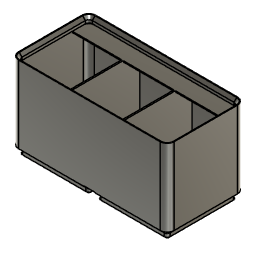
ForAnythingElse (Autodesk Fusion 360 design; units mm, degrees)
Autodesk Fusion 360 part; units mm, degrees
note: some values were not read from the file. Set by a fixed rule: which sketch regions a step uses.
ref_plane "WorkPlane9" through (0, 0, 5) normal (0, 0, 1) x (1, 0, 0)
ref_plane "WorkPlane10" through (21, 0, 0) normal (1, 0, 0) x (0, 1, 0)
ref_plane "WorkPlane11" through (0, 0, 42) normal (0, 0, 1) x (1, 0, 0)
sketch "BlockBaseProfle" plane through (0, 0, 0) normal (0, 0, 1) x (1, 0, 0)
  line L0 (0, 42) -> (42, 42)
  line L1 (42, 42) -> (42, 0)
  line L2 (42, 0) -> (0, 0)
  line L3 (0, 0) -> (0, 42)
  line L4 (0, 42) -> (42, 0) construction
  circle A0 centre (8, 8) radius 3.25
  circle A1 centre (8, 8) radius 1.5
  circle A2 centre (34, 8) radius 3.25
  circle A3 centre (34, 8) radius 1.5
  circle A4 centre (34, 34) radius 3.25
  circle A5 centre (34, 34) radius 1.5
  circle A6 centre (8, 34) radius 3.25
  circle A7 centre (8, 34) radius 1.5
  line L5 (11, 31) -> (31, 31)
  line L6 (31, 31) -> (31, 11)
  line L7 (31, 11) -> (11, 11)
  line L8 (11, 11) -> (11, 31)
  line L9 (11, 11) -> (31, 31) construction
  line L10 (4, 41.75) -> (38, 41.75)
  line L11 (41.75, 38) -> (41.75, 4)
  line L12 (38, 0.25) -> (4, 0.25)
  line L13 (0.25, 4) -> (0.25, 38)
  line L14 (21, 41.75) -> (21, 0.25) construction
  arc A8 (4, 41.75) -> (0.25, 38) centre (4, 38) ccw
  arc A9 (41.75, 38) -> (38, 41.75) centre (38, 38) ccw
  arc A10 (38, 0.25) -> (41.75, 4) centre (38, 4) ccw
  arc A11 (0.25, 4) -> (4, 0.25) centre (4, 4) ccw
  line L15 (0.25, 21) -> (41.75, 21) construction
  point P0 (21, 21)
  point P1 (21, 0.25)
  point P2 (21, 41.75)
  point P3 (0.25, 21)
  point P4 (41.75, 21)
  dimension "d8" = 42
  dimension "d11" = 8
  dimension "d12" = 8
  dimension "d13" = 6.5
  dimension "d14" = 3
  dimension "d16" = 360
  dimension "d24" = 20
  dimension "d30" = 0.25
  dimension "d31" = 3.75
  dimension "d34" = 0.25
  constraint horizontal L0
  constraint vertical L1
  constraint horizontal L2
  constraint vertical L3
  constraint equal L2 L3
  constraint midpoint L4 P0
  constraint coincident L2.end L3.start
  constraint concentric A0 A1
  constraint horizontal L5
  constraint vertical L6
  constraint horizontal L7
  constraint vertical L8
  constraint coincident L4 L6.end
  constraint coincident L4 L5.start
  constraint midpoint P0 L9
  constraint horizontal L10
  constraint vertical L11
  constraint horizontal L12
  constraint vertical L13
  constraint coincident P0 L14
  constraint coincident L10 P2
  constraint tangent L10 A8
  constraint tangent L13 A8
  constraint tangent L10 A9
  constraint tangent L11 A9
  constraint coincident L12 P1
  constraint tangent L11 A10
  constraint tangent L12 A10
  constraint equal A8 A9
  constraint tangent L12 A11
  constraint tangent L13 A11
  constraint equal A8 A11
  constraint equal A8 A10
  constraint coincident L13 P3
  constraint midpoint L11 P4
  constraint midpoint L13 P3
  constraint midpoint L14 L15
  constraint midpoint P0 L15
  constraint coincident P1 L14.end
  constraint coincident P2 L14.start
  constraint coincident P3 L15.start
  constraint coincident P4 L15.end
  measures "d8" distance of L0 L2
  measures "d11" distance of L3 A0.centre
  measures "d12" distance of L2 A0.centre
  measures "d13" diameter of A0
  measures "d14" diameter of A1
  measures "d24" distance of L5.start L5.end
  measures "d30" distance of L3 L13
  measures "d31" radius of A8
  measures "d34" distance of L0 L10
sketch "HoleSupports" plane through (0, 0, 0) normal (0, 0, 1) x (1, 0, 0)
  circle A0 centre (8, 8) radius 3.25
  circle A1 centre (8, 8) radius 1.5
  line L0 (10.8831, 9.5) -> (10.758, 9.5)
  line L1 (10.758, 9.5) -> (5.1169, 9.5)
  line L2 (10.8831, 6.5) -> (5.1169, 6.5)
  line L3 (6.5, 6.5) -> (6.5, 9.5)
  line L4 (9.5, 9.5) -> (9.5, 6.5)
  line L5 (35.5, 6.5) -> (32.5, 6.5)
  circle A2 centre (34, 8) radius 1.5
  line L6 (32.5, 9.5) -> (35.5, 9.5)
  line L7 (32.5, 10.8831) -> (32.5, 10.758)
  line L8 (32.5, 10.758) -> (32.5, 5.1169)
  circle A3 centre (34, 8) radius 3.25
  line L9 (35.5, 10.8831) -> (35.5, 5.1169)
  line L10 (35.5, 35.5) -> (35.5, 32.5)
  circle A4 centre (34, 34) radius 1.5
  line L11 (32.5, 32.5) -> (32.5, 35.5)
  line L12 (31.1169, 32.5) -> (31.242, 32.5)
  line L13 (31.242, 32.5) -> (36.8831, 32.5)
  circle A5 centre (34, 34) radius 3.25
  line L14 (31.1169, 35.5) -> (36.8831, 35.5)
  line L15 (6.5, 35.5) -> (9.5, 35.5)
  circle A6 centre (8, 34) radius 1.5
  line L16 (9.5, 32.5) -> (6.5, 32.5)
  line L17 (9.5, 31.1169) -> (9.5, 31.242)
  line L18 (9.5, 31.242) -> (9.5, 36.8831)
  circle A7 centre (8, 34) radius 3.25
  line L19 (6.5, 31.1169) -> (6.5, 36.8831)
  point P0 (21, 21)
  dimension "d113" = 360
  constraint coincident A0 L0.start
  constraint horizontal L0
  constraint coincident A0 L1.end
  constraint parallel L0 L1
  constraint coincident A0 L2.start
  constraint coincident A0 L2.end
  constraint parallel L1 L2
  constraint coincident L2 L3.start
  constraint coincident L1 L3.end
  constraint perpendicular L1 L3
  constraint coincident L1 L4.start
  constraint perpendicular L1 L4
  constraint tangent A1 L1
  constraint tangent A1 L2
  constraint tangent A1 L3
  constraint tangent A1 L4
  constraint coincident L2 L4.end
sketch "BlockMaskProfile" plane through (0, 0, 0) normal (0, 0, 1) x (1, 0, 0)
  line L0 (4, 41.75) -> (80, 41.75)
  line L1 (83.75, 38) -> (83.75, 4)
  line L2 (80, 0.25) -> (4, 0.25)
  line L3 (0.25, 4) -> (0.25, 38)
  arc A0 (0.25, 4) -> (4, 0.25) centre (4, 4) ccw
  arc A1 (80, 0.25) -> (83.75, 4) centre (80, 4) ccw
  arc A2 (83.75, 38) -> (80, 41.75) centre (80, 38) ccw
  arc A3 (4, 41.75) -> (0.25, 38) centre (4, 38) ccw
  line L4 (42, 0.25) -> (42, 41.75) construction
  line L5 (0.25, 21) -> (83.75, 21) construction
  line L6 (84, 0) -> (0, 0)
  line L7 (0, 0) -> (0, 42)
  line L8 (0, 42) -> (84, 42)
  line L9 (84, 42) -> (84, 0)
  line L10 (126, -42) -> (-42, -42)
  line L11 (-42, -42) -> (-42, 84)
  line L12 (-42, 84) -> (126, 84)
  line L13 (126, 84) -> (126, -42)
  arc A4 (1.05, 4) -> (4, 1.05) centre (4, 4) ccw
  line L14 (80, 1.05) -> (4, 1.05)
  arc A5 (80, 1.05) -> (82.95, 4) centre (80, 4) ccw
  line L15 (82.95, 38) -> (82.95, 4)
  arc A6 (82.95, 38) -> (80, 40.95) centre (80, 38) ccw
  line L16 (4, 40.95) -> (80, 40.95)
  arc A7 (4, 40.95) -> (1.05, 38) centre (4, 38) ccw
  line L17 (1.05, 4) -> (1.05, 38)
  dimension "d54" = 3.75
  dimension "d56" = 41.5
  dimension "d57" = 83.5
  dimension "d61" = 0.25
  dimension "d62" = 0.25
  dimension "d63" = 0.25
  dimension "d64" = 0.25
  dimension "d154" = 42
  dimension "d155" = 42
  dimension "d232" = 42
  dimension "d315" = 0.8
  constraint horizontal L0
  constraint vertical L1
  constraint horizontal L2
  constraint vertical L3
  constraint tangent L2 A0
  constraint tangent L3 A0
  constraint tangent L1 A1
  constraint tangent L2 A1
  constraint equal A0 A1
  constraint tangent L0 A2
  constraint tangent L1 A2
  constraint equal A0 A2
  constraint tangent L0 A3
  constraint tangent L3 A3
  constraint equal A0 A3
  constraint midpoint L2 L4.start
  constraint midpoint L0 L4.end
  constraint midpoint L3 L5.start
  constraint midpoint L1 L5.end
  constraint horizontal L6
  constraint vertical L7
  constraint horizontal L8
  constraint vertical L9
  constraint coincident L6.end L7.start
  constraint horizontal L10
  constraint vertical L11
  constraint horizontal L12
  constraint vertical L13
  measures "d54" radius of A0
  measures "d56" distance of L4.start L4.end
  measures "d57" distance of L5.start L5.end
  measures "d61" distance of L3 L7
  measures "d62" distance of L1 L9
  measures "d63" distance of L2 L6
  measures "d64" distance of L0 L8
  measures "d154" distance of L9 L13
  measures "d155" distance of L7 L11
  measures "d232" distance of L8.end L12
sketch "NestingProfile" plane through (21, 0, 0) normal (1, 0, 0) x (0, 1, 0)
  line L0 (0, 0) -> (-5, 0)
  line L1 (-5, 0) -> (-5, 7)
  line L2 (0, 5) -> (0, 0) construction
  line L3 (0, 5) -> (2.4, 2.6)
  line L4 (2.4, 2.6) -> (2.4, 0.8)
  line L5 (2.4, 0.8) -> (3.2, 0)
  line L6 (3.2, 0) -> (0, 0)
  line L7 (1.05, 5.0814) -> (5.3314, 0.8)
  line L8 (5.3314, 0.8) -> (21, 0.8)
  line L9 (21, 0) -> (21, 5)
  line L10 (0, 5) -> (0, 7)
  line L11 (0, 7) -> (-5, 7)
  line L12 (1.05, 5.0814) -> (1.05, 7)
  line L13 (1.05, 7) -> (21, 7)
  line L14 (21, 7) -> (21, 5)
  line L15 (1.05, 5.8) -> (0, 5.8) construction
  line L16 (1.05, 5.0814) -> (0.3314, 5.8)
  line L17 (0.3314, 5.8) -> (0.3314, 7)
  line L18 (0.3314, 7) -> (1.05, 7)
  line L19 (0.6464, 46) -> (2.15, 44.4964)
  line L20 (2.4, 44.6) -> (2.4, 42.8) construction
  line L21 (1.05, 41.8964) -> (0.25, 41.8964)
  line L22 (0.6464, 46) -> (0.25, 46)
  line L23 (2.15, 44.4964) -> (2.15, 42.9964)
  line L24 (2.15, 42.9964) -> (1.05, 41.8964)
  line L25 (0.25, 46.75) -> (2.4, 44.6) construction
  line L26 (0.25, 41.8964) -> (0.25, 46.75)
  line L27 (13.8368, 42) -> (0.4771, 42)
  point P0 (0.25, 0)
  point P1 (21, 0)
  point P2 (0.25, 42)
  dimension "d36" = 45
  dimension "d37" = 2.4
  dimension "d38" = 0.8
  dimension "d39" = 1.8
  dimension "d65" = 0.8
  dimension "d97" = 45
  dimension "d98" = 2
  dimension "d99" = 5
  dimension "d133" = 1.05
  dimension "d134" = 0.8
  dimension "d200" = 5
  dimension "d313" = 0.8
  dimension "d316" = 45
  dimension "d317" = 2.15
  dimension "d318" = 1.8
  dimension "d319" = 0.8
  dimension "d320" = 0.25
  dimension "d321" = 0.25
  dimension "d346" = 45
  dimension "d347" = 0.8
  dimension "d362" = 4
  dimension "d363" = 1.5
  dimension "d326" = 0.25
  constraint horizontal L0
  constraint perpendicular L0 L1
  constraint vertical L2
  constraint parallel L3 L5
  constraint perpendicular L2 L6
  constraint coincident L0.start L2.end
  constraint parallel L3 L7
  constraint perpendicular L2 L8
  constraint coincident P1 L9.start
  constraint vertical L9
  constraint coincident L9 L14.end
  constraint perpendicular L10 L11
  constraint perpendicular L1 L11
  constraint perpendicular L12 L13
  constraint perpendicular L13 L14
  constraint horizontal L10.end L12.end
  constraint parallel L10 L12
  constraint coincident L12 L15.start
  constraint coincident L10 L15.end
  constraint perpendicular L10 L15
  constraint coincident L15 L16.end
  constraint collinear L7 L16
  constraint perpendicular L15 L17
  constraint perpendicular L17 L18
  constraint vertical L26
  constraint parallel L20 L26
  constraint perpendicular L21 L26
  constraint coincident L22.end L26
  constraint perpendicular L22 L26
  constraint coincident L24.start L23
  constraint coincident P2 L26
  constraint horizontal P2 L27.end
  measures "d36" angle of L3 L4
  measures "d37" horizontal distance of L2.start L3.end
  measures "d38" horizontal distance of L4.end L5.end
  measures "d39" distance of L3.end L4.end
  measures "d65" distance of L8 P1
  measures "d97" angle of L3 L10
  measures "d98" distance of L2.start L10.end
  measures "d99" distance of L0.end L0.start
  measures "d133" distance of L10.end L12.end
  measures "d134" distance of L3 L7
  measures "d200" distance of L0.start L2.start
  measures "d313" distance of L2.start L15
  measures "d316" angle of L25 L26
  measures "d317" vertical distance of L20.start L25.start
  measures "d318" distance of L20.start L20.end
  measures "d319" distance of L21.end L21.start
  measures "d320" distance of L19 L25
  measures "d321" distance of L20 L23
  measures "d346" angle of L21 L24
  measures "d347" vertical distance of P2 L20.end
  measures "d362" distance of L22.end P2
  measures "d363" distance of L19.end L23.end
  measures "d326" horizontal distance of L10.end P2
extrude "Extrude1" add sketch "BlockBaseProfle" along normal up to surface (5.8 mm away) contours L0 L1 L2 L3 | A0 | A1 | A2 | A3 | A4 | A5 | A6 | A7 | L5 L6 L7 L8 | L10 L11 L12 L13 A8 A9 A10 A11 makes body 1 in component "Block_Base"
sweep "Sweep1" cut profiles "NestingProfile" path "BlockBaseProfle" along L12 A10 L11 A9 L10 A8 L13 A11 section 1 contours L0 L1 L3 L4 L5 L6 L10 L11 bodies 1 in component "Block_Base"
extrude "WeightPocket" [suppressed] in component "Block_Base"
pattern_linear "R-Pattern1" count 2 spacing 42 along (1, 0, 0) of bodies 1 makes body 2 in component "Block_Base"
extrude "Extrude20" add sketch "BlockMaskProfile" along normal blind 0.8 from surface at 5 contours L0 L1 L2 L3 A0 A1 A2 A3 | A4 L14 A5 L15 A6 L16 A7 L17 bodies 1 2 in component "Block_Base"
extrude "Extrude7" cut sketch "BlockMaskProfile" along normal blind 59 contours L6 L7 L8 L9 | L10 L11 L12 L13 bodies 1 in component "Block_Base"
extrude "Extrude3" add sketch "BlockMaskProfile" along normal up to surface (5.8 mm away) separate body contours L0 L1 L2 L3 A0 A1 A2 A3 | L6 L7 L8 L9 | L10 L11 L12 L13 | A4 L14 A5 L15 A6 L16 A7 L17 makes body 3
combine "Combine2" operation cut target body 3 tool bodies 1 keep tools
extrude "Extrude4" add 1 faces at (54.6667, 69.9167, 5.8) along direction (0, 0, 1) blind 42 on bodies 3 bodies 3
extrude "Extrude25" add sketch "BlockMaskProfile" along normal up to surface (37 mm away) from surface at 5 contours L0 L1 L2 L3 A0 A1 A2 A3 bodies 1 in component "Block_Base"
sweep "Sweep8" add profiles "NestingProfile" path "BlockMaskProfile" along L1 A2 L0 A3 L3 A0 L2 A1 section 1 contours L19 L21 L22 L23 L24 L26 bodies 1 in component "Block_Base"
sketch "ScoopProfile" plane through (21, 0, 0) normal (1, 0, 0) x (0, 1, 0) in component "Block_Base"
  arc A0 (2.15, 15.8) -> (12.15, 5.8) centre (12.15, 15.8) ccw
  arc A1 (1.35, 15.8) -> (5.9554, 6.9532) centre (12.15, 15.8) ccw
  line L0 (1.35, 42.9964) -> (1.35, 15.8)
  line L1 (5.9554, 6.9532) -> (7.6023, 5.8)
  line L2 (4, 5.8) -> (20.7133, 5.8)
  line L3 (80, 5.8) -> (4, 5.8)
  line L4 (2.15, 42.9964) -> (2.15, 15.8)
  line L5 (1.35, 42.9964) -> (2.15, 42.9964)
  point P0 (0.25, 67.3684)
  point P1 (4, 5.8)
  point P2 (2.15, 42.9964)
  dimension "d260" = 10
  dimension "d268" = 35
  dimension "d333" = 0.8
  constraint tangent A1 L0
  constraint tangent A1 L1
  constraint concentric A0 A1
  constraint coincident A0.end L2
  constraint tangent A0 L2
  constraint horizontal L2
  constraint coincident L2 P1
  constraint coincident P1 L2.start
  constraint coincident L1.end L2
  constraint coincident P2 L4.start
  constraint tangent A0 L4
  constraint vertical L4
  constraint vertical L0
  constraint perpendicular L4 L5
  measures "d260" radius of A0
  measures "d268" angle of L1 L2
  measures "d333" distance of L0.start P2
extrude "Extrude27" add sketch "ScoopProfile" along normal up to surface (-20.75 mm away) and the other way up to surface (-62.75 mm away) bodies 1 in component "Block_Base"
sketch "ScoopDividers" plane through (0, 0, 42) normal (0, 0, 1) x (1, 0, 0)
  line L0 (27.6, 0) -> (28.4, 0)
  line L1 (28.4, 0) -> (28.4, 42)
  line L2 (28.4, 42) -> (27.6, 42)
  line L3 (27.6, 42) -> (27.6, 0)
  line L4 (28, 0) -> (28, 42) construction
  dimension "d282" = 0.8
  dimension "d283" = 42
  dimension "d284" = 28
  constraint horizontal L0
  constraint vertical L1
  constraint horizontal L2
  constraint vertical L3
  constraint horizontal L0.start origin
  constraint midpoint L0 L4.start
  constraint midpoint L2 L4.end
  measures "d282" distance of L1 L3
  measures "d283" distance of L0.start L2.end
  measures "d284" distance of origin L4
extrude "Extrude28" add sketch "ScoopDividers" against normal up to surface (42 mm away) bodies 1 in component "Block_Base"
pattern_linear "R-Pattern6" count 2 spacing 28 along (1, 0, 0) of "Extrude28" in component "Block_Base"
sketch "FullLabel" plane through (0, 0, 42) normal (0, 0, 1) x (1, 0, 0)
  line L0 (84, 32) -> (0, 32)
  line L1 (0, 32) -> (0, 42)
  line L2 (0, 42) -> (84, 42)
  line L3 (84, 42) -> (84, 32)
  dimension "d291" = 10
  dimension "d292" = 84
  dimension "d293" = 42
  constraint horizontal L0
  constraint vertical L1
  constraint horizontal L2
  constraint vertical L3
  constraint vertical origin L1.end
  measures "d291" distance of L0 L2
  measures "d292" distance of L1.end L2.end
  measures "d293" distance of origin L1.end
sketch "LabelSupports" plane through (21, 0, 0) normal (1, 0, 0) x (0, 1, 0)
  line L0 (42, 42) -> (32, 42)
  line L1 (42, 35.6265) -> (42, 42)
  line L2 (32, 42) -> (32, 41.4)
  line L3 (32, 41.4) -> (42, 35.6265)
  dimension "d297" = 0.6
  dimension "d298" = 60
  constraint coincident L0.start L1.end
  constraint perpendicular L0 L1
  constraint coincident L0.end L2.start
  constraint perpendicular L0 L2
  measures "d297" distance of L0.end L2.end
  measures "d298" angle of L1 L3
sketch "Sketch12" plane through (0, 0, 42) normal (0, 0, 1) x (1, 0, 0)
  line L0 (0, 42) -> (84, 42)
sweep "Sweep9" add profiles "LabelSupports" path "Sketch12" along L0 section 1 bodies 1 in component "Block_Base"
extrude "Extrude29" [suppressed] in component "Block_Base"
extrude "Extrude30" [suppressed] in component "Block_Base"
pattern_linear "R-Pattern7" [suppressed] in component "Block_Base"
extrude "Extrude31" [suppressed] in component "Block_Base"
pattern_linear "R-Pattern8" [suppressed] in component "Block_Base"
combine "Combine2'" operation cut target body 1 tool bodies 3 keep tools in component "Block_Base"
component "Block_Base" placed x (1, 0, 0) y (0, 1, 0) z (0, 0, 1) at (0, 0, 0)
equation "SU_Height = 7 mm"
equation "SlotsDeep = 1"
equation "SlotsWide = 2"
equation "SU_Slot = 42 mm"
equation "PR_LayerHeight = 0.2 mm"
equation "PR_WallThickness = 0.8 mm"
equation "d8 = SU_Slot"
equation "MagnetDiameter = 6.5 mm"
equation "ScrewDiameter = 3 mm"
equation "d12 = d11"
equation "d13 = MagnetDiameter"
equation "d14 = ScrewDiameter"
equation "NestingDepth = 5 mm"
equation "NestingRimWidth = 2.4 mm"
equation "NestingClearance = 0.25 mm"
equation "CornerFillet = 4 mm"
equation "MagnetThickness = 2.4 mm"
equation "WeightSlot = 20 mm"
equation "WeightDepth = 4 mm"
equation "d24 = WeightSlot"
equation "WallThickness = 1.2 mm"
equation "d30 = NestingClearance"
equation "d31 = CornerFillet - NestingClearance"
equation "d34 = d30"
equation "UHeight = 6"
equation "d50 = SlotsWide"
equation "d51 = SlotsDeep"
equation "d52 = SU_Slot"
equation "d53 = SU_Slot"
equation "d54 = CornerFillet - NestingClearance"
equation "d56 = ( SlotsDeep * SU_Slot ) - ( NestingClearance * 2 )"
equation "d57 = ( SlotsWide * SU_Slot ) - ( NestingClearance * 2 )"
equation "d61 = NestingClearance"
equation "d62 = NestingClearance"
equation "d63 = NestingClearance"
equation "d64 = NestingClearance"
equation "d133 = PR_WallThickness + NestingClearance"
equation "d135 = WeightDepth"
equation "MaxScoopRadius = 10 mm" comment "Max 18.85"
equation "Scoop = min(MaxScoopRadius; ( ( SU_Height * UHeight ) / 2 ))"
equation "d154 = SU_Slot"
equation "d155 = d154"
equation "DividerSpacing_Wide = ( SlotsWide * SU_Slot ) / DividerWide_Count"
equation "DividerWide_Count = 3"
equation "d197 = NestingDepth"
equation "d198 = PR_WallThickness"
equation "d229 = NestingDepth"
equation "d230 = SU_Slot / 2"
equation "d231 = SU_Height * UHeight"
equation "d232 = SU_Slot"
equation "d233 = PR_WallThickness"
equation "d260 = Scoop"
equation "d273 = PR_WallThickness"
equation "d275 = SU_Height * UHeight"
equation "d282 = PR_WallThickness"
equation "d283 = SU_Slot * SlotsDeep"
equation "d284 = DividerSpacing_Wide"
equation "d287 = DividerWide_Count - 1"
equation "d289 = DividerSpacing_Wide"
equation "d292 = SU_Slot * SlotsWide"
equation "d293 = SU_Slot * SlotsDeep"
equation "d294 = -PR_LayerHeight * 3"
equation "d297 = PR_LayerHeight * 3"
equation "d299 = PR_WallThickness"
equation "d301 = SlotsWide"
equation "d303 = SU_Slot"
equation "d305 = SU_Slot / 2"
equation "d306 = PR_WallThickness"
equation "d308 = SlotsWide - 1"
equation "d310 = -SU_Slot"
equation "d313 = PR_WallThickness"
equation "d314 = NestingDepth"
equation "d315 = PR_WallThickness"
equation "d319 = PR_WallThickness"
equation "d326 = NestingClearance"
equation "d333 = PR_WallThickness"
named bodies: "CutMask"
